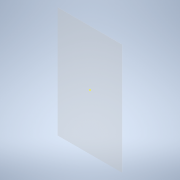
# Autodesk Inventor part: acrilico
Saved by Autodesk Inventor 2021.2 (Build 252289000, 289)
## iProperties
Created: 2026-06-02
Part Number: acrilico
Material: Cristal
Document SubType Name: Modeling
Designer: nelso
Density: 2.18 g/cm^3
Appearance: Transparente - Claro
Mass: 9370.9 g
Surface Area: 28808.3 cm^2
Volume: 4298.58 cm^3
Author: nelso
Autodesk Inventor part; units mm, degrees
ref_plane "YZ Plane" through (0, 0, 0) normal (1, 0, 0) x (0, 1, 0)
ref_plane "XZ Plane" through (0, 0, 0) normal (0, 1, 0) x (-1, 0, 0)
ref_plane "XY Plane" through (0, 0, 0) normal (0, 0, 1) x (1, 0, 0)
sketch "Sketch1" plane through (0, 0, 0) normal (0, 0, 1) x (1, 0, 0)
  line L0 (-434.2, -825) -> (434.2, -825)
  line L1 (434.2, -825) -> (434.2, 825)
  line L2 (434.2, 825) -> (-434.2, 825)
  line L3 (-434.2, 825) -> (-434.2, -825)
  line L4 (-434.2, -825) -> (434.2, 825) construction
  line L5 (434.2, -825) -> (-434.2, 825) construction
  point P0 (0, 0)
  dimension "d0" = 868.4
  dimension "d1" = 1650
  constraints: 12 end point, 2 midpoint, 2 parallel, 1 horizontal, 1 perpendicular
  measures "d0" distance of L2.end L1.end
  measures "d1" distance of L1.end L0.end
extrude "Extrusion1" add sketch "Sketch1" along normal blind 3
sketch "Sketch2" plane through (0, 0, 3) normal (0, 0, 1) x (1, 0, 0)
  point P0 (0, 0)
body "Solid1"
